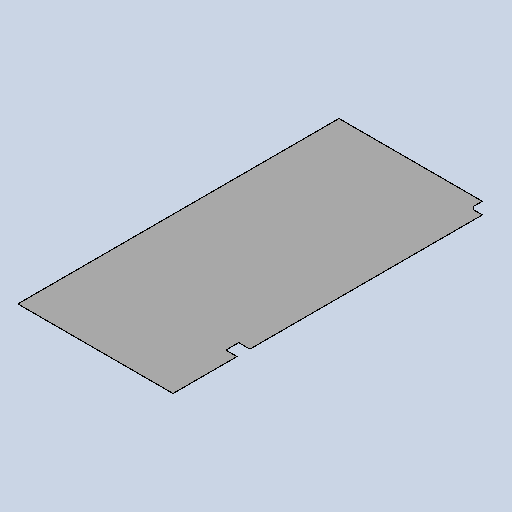
# Autodesk Inventor part: PNS-0113 floor sheet 3
Saved by Autodesk Inventor 2025.1 (Build 291241020, 241B)
## iProperties
Created: 2025-03-10
Part Number: PNS-0113 floor sheet 3
Material: Stainless Steel
Description: DIE16(5)|\ 90°|corrY -___°|X_____|bom___
Document SubType Name: Sheet Metal
Designer: user
Stock Number: МОО 305 шпангоут борт
Mass: 72000 g
Surface Area: 90180 cm^2
Volume: 9000 cm^3
Density: 8 g/cm^3
Sheet Metal Rule: AISI304 2mm Die16
Sheet Metal Width: 0.000 mm
Sheet Metal Length: 0.000 mm
Sheet Metal Area: 0.000 mm^2
Appearance: Default
Author: admin
Autodesk Inventor part; units mm, degrees
ref_plane "YZ Plane" through (0, 0, 0) normal (1, 0, 0) x (0, 1, 0)
ref_plane "XZ Plane" through (0, 0, 0) normal (0, 1, 0) x (-1, 0, 0)
ref_plane "XY Plane" through (0, 0, 0) normal (0, 0, 1) x (1, 0, 0)
sketch "Sketch1" plane through (0, 0, 0) normal (0, 0, 1) x (1, 0, 0)
  line L0 (-722.5, -1495) -> (722.5, -1495)
  line L1 (722.5, -1495) -> (722.5, 1495)
  line L2 (722.5, 1495) -> (-722.5, 1495)
  line L3 (-722.5, 1495) -> (-722.5, -1495)
  line L4 (-722.5, -1495) -> (722.5, 1495) construction
  line L5 (722.5, -1495) -> (-722.5, 1495) construction
  line L6 (722.5, -779) -> (618.5, -779)
  line L7 (618.5, -779) -> (618.5, -899)
  line L8 (618.5, -899) -> (722.5, -899)
  line L9 (722.5, -899) -> (722.5, -779)
  line L10 (722.5, 1385) -> (612.5, 1385)
  line L11 (612.5, 1385) -> (612.5, 1495)
  point P0 (0, 0)
  point P1 (722.5, -899)
  dimension "d154" = 1445
  dimension "d155" = 2990
  dimension "d159" = 120
  dimension "d161" = 104
  dimension "d162" = 596
  dimension "d163" = 110
  measures "d154" distance of L1.end L2.end
  measures "d155" distance of L0.end L1.end
  measures "d159" distance of L6.end L7.end
  measures "d161" distance of L7.end L8.end
  measures "d162" distance between parallel lines of L0 L8
  measures "d163" distance of L10.start L10.end
extrude "Plate5" add sketch "Sketch1" along normal blind 2 contours L3 L2 L11 L10 L1 L6 L7 L8 L0
chamfer "Corner Chamfer2" distance 30 angle 45 1 edges at (612.5, 1385, 1)
body "Solid3"
